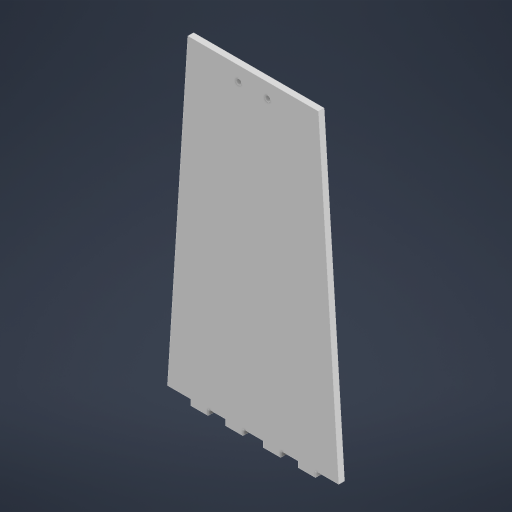
# Autodesk Inventor part: Langbektang houder
Saved by Autodesk Inventor 2023.2 (Build 272271000, 271)
## iProperties
Created: 2020-09-09
Part Number: Langbektang houder
Material: Generic
Document SubType Name: Modeling
Designer: nathan.bollaert
Density: 1 g/cm^3
Appearance: Default
Author: nathan.bollaert
Autodesk Inventor part; units mm, degrees
ref_plane "YZ Plane" through (0, 0, 0) normal (1, 0, 0) x (0, 1, 0)
ref_plane "XZ Plane" through (0, 0, 0) normal (0, 1, 0) x (-1, 0, 0)
ref_plane "XY Plane" through (0, 0, 0) normal (0, 0, 1) x (1, 0, 0)
sketch "Sketch1" plane through (0, 0, 0) normal (0, 0, 1) x (1, 0, 0)
  line L0 (0, 0) -> (14, 215.5374)
  line L1 (14, 215.5374) -> (104, 215.5374)
  line L2 (104, 215.5374) -> (118, 0)
  line L3 (16, 0) -> (28, 0)
  line L4 (28, 0) -> (28, -4)
  line L5 (28, -4) -> (16, -4)
  line L6 (16, -4) -> (16, 0)
  line L7 (66, 0) -> (78, 0)
  line L8 (78, 0) -> (78, -4)
  line L9 (78, -4) -> (66, -4)
  line L10 (66, -4) -> (66, 0)
  line L11 (40, 0) -> (52, 0)
  line L12 (52, 0) -> (52, -4)
  line L13 (52, -4) -> (40, -4)
  line L14 (40, -4) -> (40, 0)
  line L15 (90, 0) -> (102, 0)
  line L16 (102, 0) -> (102, -4)
  line L17 (102, -4) -> (90, -4)
  line L18 (90, -4) -> (90, 0)
  line L19 (78, 0) -> (90, 0)
  line L20 (28, 0) -> (40, 0)
  line L21 (102, 0) -> (118, 0)
  line L22 (16, 0) -> (0, 0)
  line L23 (52, 0) -> (66, 0)
  line L24 (102, -4) -> (118.2598, -4)
  line L25 (118.2598, -4) -> (118, 0)
  dimension "d229" = 90
  dimension "d232" = 16
  dimension "d233" = 12
  dimension "d234" = 12
  dimension "d235" = 4
  dimension "d239" = 14
  dimension "d241" = 220
  constraints: 52 end point, 9 equal length, 9 horizontal, 8 parallel, 4 perpendicular, 3 collinear
  measures "d229" distance of L0.end L1.end
  measures "d232" horizontal distance of L0.start L5.end
  measures "d233" distance of L4.end L5.end
  measures "d234" distance of L3.end L11.start
  measures "d235" distance of L5.end L3.start
  measures "d239" distance between parallel lines of L10 L12
  measures "d241" distance of L24.end L1.end
extrude "Extrusion1" add sketch "Sketch1" against normal blind 4 contours L0 L1 L2 L21 L15 L19 L7 L23 L11 L20 L3 L22 | L3 L4 L5 L6 | L11 L12 L13 L14 | L16 L17 L18 L15 | L7 L8 L9 L10
sketch "Sketch2" plane through (0, 0, 0) normal (0, 0, 1) x (1, 0, 0)
  circle A0 centre (49, 205.5374) radius 2
  circle A1 centre (69, 205.5374) radius 2
  line L0 (104, 215.5374) -> (14, 215.5374) projected
  line L1 (14, 215.5374) -> (104, 215.5374) projected
  line L2 (59, 215.5374) -> (59, 0)
  line L3 (52, 0) -> (66, 0) projected
  point P0 (0, 0)
  dimension "d242" = 4
  dimension "d244" = 10
  dimension "d245" = 20
  constraints: 2 centre point, 2 end point, 2 midpoint, 1 equal radius, 1 horizontal alignment, 1 other
  measures "d242" diameter of A0
  measures "d244" distance from line of L0 A0.centre
  measures "d245" distance of A0.centre A1.centre
extrude "Extrusion17" cut sketch "Sketch2" against normal blind 4
body "Solid5"
